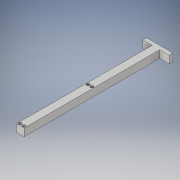
# Autodesk Inventor part: new cup 2
Saved by Autodesk Inventor 2017.3 (Build 213256000, 256)
## iProperties
Created: 2018-08-30
Part Number: new cup 2
Material: Generic
Document SubType Name: Modeling
Designer: Mac
Density: 1 g/cm^3
Appearance: Default
Author: Mac
Autodesk Inventor part; units mm, degrees
ref_plane "YZ Plane" through (0, 0, 0) normal (1, 0, 0) x (0, 1, 0)
ref_plane "XZ Plane" through (0, 0, 0) normal (0, 1, 0) x (-1, 0, 0)
ref_plane "XY Plane" through (0, 0, 0) normal (0, 0, 1) x (1, 0, 0)
sketch "Sketch1" plane through (0, 0, 0) normal (0, 0, 1) x (1, 0, 0)
  line L0 (0, 0) -> (-22.225, 0)
  line L1 (-22.225, 0) -> (-22.225, 6.35)
  line L2 (-22.225, 6.35) -> (0, 6.35)
  line L3 (0, 6.35) -> (0, 0)
  dimension "d0" = 22.225
  dimension "d1" = 6.35
  constraints: 8 end point, 2 parallel, 1 horizontal, 1 perpendicular
  measures "d0" distance of L1.end L2.end
  measures "d1" distance of L0.end L1.end
extrude "Extrusion1" add sketch "Sketch1" along normal blind 3.175
sketch "Sketch2" plane through (0, 0, 3.175) normal (0, 0, 1) x (1, 0, 0)
  line L0 (0, 6.35) -> (-22.225, 6.35) projected
  line L1 (-7.9375, 6.35) -> (-14.2875, 6.35)
  line L2 (-14.2875, 6.35) -> (-14.2875, 0)
  line L3 (-14.2875, 0) -> (-7.9375, 0)
  line L4 (-7.9375, 0) -> (-7.9375, 6.35)
  point P0 (0, 0)
  dimension "d4" = 6.35
  constraints: 8 end point, 2 parallel, 1 horizontal, 1 perpendicular, 1 point on line
  measures "d4" distance of L3.end L2.end
extrude "Extrusion2" add sketch "Sketch2" along normal blind 114.3
sketch "Sketch3" plane through (-22.225, 6.35, 0) normal (0, 1, 0) x (1, 0, 0)
  point P0 (22.225, 0)
  point P1 (9.5377, -115.8875)
  point P2 (12.7127, -115.9002)
  point P3 (9.5377, -58.7502)
  point P4 (12.7254, -58.7502)
hole "Hole1" at (-12.6873, 6.35, 115.8875) at (-9.5123, 6.35, 115.9002) at (-12.6873, 6.35, 58.7502) at (-9.4996, 6.35, 58.7502) direction (0, -1, 0) diameter 2.4892 depth 9.525 tip angle 118
body "Solid1"
